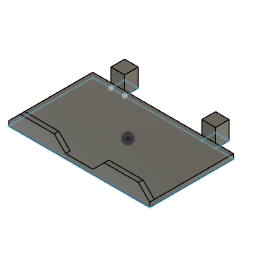
secondary_015mm_cover (Autodesk Fusion 360 design; units mm, degrees)
Autodesk Fusion 360 part; units mm, degrees
other "Base Mesh Feature1"
sketch "Sketch1" plane through (0, 0, 0) normal (0, 0, 1) x (1, 0, 0)
  circle A0 centre (0, 0) radius 1
  dimension "d1" = 2
  constraint coincident A0.centre origin
  measures "d1" diameter of A0
other "Modify1"
sketch "Sketch2" plane through (0, 0, 0) normal (0, 0, 1) x (1, 0, 0)
  line L0 (30.9937, -21.4361) -> (-31.0349, -21.4361)
  line L1 (-31.0349, -21.4361) -> (-31.0349, 15.4994)
  line L2 (30.9937, 15.4994) -> (30.9937, -21.4361)
  line L3 (23, 15.4994) -> (17.0002, 15.4994)
  line L4 (17.0002, 15.4994) -> (17.0002, 21.4994)
  line L5 (17.0002, 21.4994) -> (23, 21.4994)
  line L6 (23, 21.4994) -> (23, 15.4994)
  line L7 (-22.9998, 15.4994) -> (-22.9998, 21.4994)
  line L8 (-22.9998, 21.4994) -> (-17, 21.4994)
  line L9 (-17, 21.4994) -> (-17, 15.4994)
  line L10 (-31.0349, 15.4994) -> (17.0002, 15.4994)
  line L11 (23, 15.4994) -> (30.9937, 15.4994)
  constraint horizontal L0
  constraint vertical L1
  constraint horizontal L10
  constraint vertical L2
  constraint horizontal L3
  constraint vertical L4
  constraint horizontal L5
  constraint vertical L6
  constraint coincident L3.start L10
  constraint vertical L7
  constraint horizontal L8
  constraint vertical L9
  constraint collinear L10 L11
extrude "Extrude1" add sketch "Sketch2" along normal blind 2 contours L0 L1 L2 L3 L10 L11 makes body 1
extrude "Extrude2" add sketch "Sketch2" along normal blind 8 separate body contours L3 L4 L5 L6 | L7 L8 L9 L10 makes body 2 at (17.0002, 17.4994, 2.6667) makes body 3 at (-22.9998, 17.4994, 2.6667)
sketch "Sketch3" plane through (0, -21.4361, 0) normal (0, -1, 0) x (1, 0, 0)
  line L0 (-31.0349, 0) -> (30.9937, 0)
  line L1 (30.9937, 0) -> (30.9937, 2)
  line L2 (30.9937, 2) -> (-31.0349, 2)
  line L3 (-31.0349, 2) -> (-31.0349, 0)
  line L4 (-31.0349, 2) -> (-26, 7)
  line L5 (-26, 7) -> (-11, 7)
  line L6 (-11, 7) -> (-6.0347, 2)
  line L7 (30.9937, 2) -> (26.0284, 7)
  line L8 (26.0284, 7) -> (11, 7)
  line L9 (11, 7) -> (6, 2)
  constraint coincident L2.end L3.start
  constraint perpendicular L3 L5
  constraint coincident L2 L6.end
  constraint perpendicular L4 L6
  constraint coincident L1.end L2.start
  constraint parallel L6 L7
  constraint perpendicular L1 L8
  constraint coincident L2 L9.end
extrude "Extrude3" add sketch "Sketch3" against normal blind 2 contours L2 L4 L5 L6 | L2 L7 L8 L9 bodies 1
combine "Combine1" operation add target body 1 tool bodies 2 3
copy_body "Body->Comp1" bodies 1 removing the originals makes body 4 in component "secondary_015mm_cover"
component "secondary_015mm_cover" placed x (1, 0, 0) y (0, 1, 0) z (0, 0, 1) at (0, 0, 0)
named bodies: "secondary_015mm_cover (1)"
